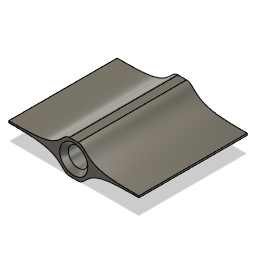
hose_to_balloon_symmetrical v2 (Autodesk Fusion 360 design; units mm, degrees)
Autodesk Fusion 360 part; units mm, degrees
sketch "Sketch1" plane through (0, 0, 0) normal (0, 0, 1) x (1, 0, 0)
  line L0 (15, -3.85) -> (-15, -3.85)
  line L1 (-15, -3.85) -> (-15, 3.85)
  line L2 (-15, 3.85) -> (15, 3.85)
  line L3 (15, 3.85) -> (15, -3.85)
  line L4 (15, -3.85) -> (-15, 3.85) construction
  line L5 (-15, -3.85) -> (15, 3.85) construction
  circle A0 centre (0, 0) radius 2.25
  line L6 (0, 2.25) -> (0, 3.85)
  dimension "d1" = 30
  dimension "d2" = 4.5
  dimension "d3" = 1.6
  constraint horizontal L0
  constraint perpendicular L0 L1
  constraint parallel L0 L2
  constraint parallel L1 L3
  constraint coincident L4 A0.centre
  constraint coincident L5 A0.centre
  constraint coincident A0.centre origin
  constraint coincident A0 L6.start
  constraint midpoint L2 L6.end
  constraint vertical L6
  measures "d1" distance of L0.start L0.end
  measures "d2" diameter of A0
  measures "d3" vertical distance of L6.start L6.end
extrude "Extrude1" add sketch "Sketch1" along normal blind 25
sketch "Sketch2" plane through (0, 0, 25) normal (0, 0, 1) x (1, 0, 0)
  circle A0 centre (0, 0) radius 2.25
  line L0 (15, 3.85) -> (-15, 3.85)
  line L1 (-15, 3.85) -> (-15, -3.85)
  line L2 (-15, -3.85) -> (15, -3.85)
  line L3 (15, -3.85) -> (15, 3.85)
  line L4 (-15, 0) -> (0, 0)
  line L5 (0, 0) -> (0, 3.85)
  line L6 (-15, 0.2) -> (-7, 0.2)
  line L7 (-7, 0.2) -> (-3.0262, 0.3362)
  line L8 (-3.0262, 0.3362) -> (-3, 3.85)
  line L9 (-3, 3.85) -> (-1, 3.85)
  spline S0 degree 4 poles (-15, 0.2) (-7, 0.2) (-3.0262, 0.3362) (-3, 3.85) (-1, 3.85) knots 0 0 0 0 0 1 1 1 1 1
  line L10 (-1, 3.85) -> (0, 3.85)
  dimension "d6" = 8
  dimension "d7" = 0.4
  dimension "d9" = 2
  dimension "d19" = 2
  constraint midpoint L1 L4.start
  constraint coincident A0.centre L4.end
  constraint midpoint L0 L5.end
  constraint coincident L1 L6.start
  constraint coincident L0 L8.end
  constraint horizontal L6
  constraint coincident L0 L9.end
  measures "d6" distance of L6.start L6.end
  measures "d9" distance of L8.end L9.end
extrude "Extrude2" cut sketch "Sketch2" against normal through all contours L0 L8 L9 S0 | L0 L1 L8 S0
mirror "Mirror1" about plane through (0, 0, 0) normal (0, 1, 0) of "Extrude2"
mirror "Mirror2" about plane through (0, 0, 0) normal (1, 0, 0) of "Extrude2", "Mirror1"
chamfer "Chamfer1" distance 1 angle 45 1 edges at (-2.0977, 0.8136, 25)
hole "Hole1" at (0, 0, 0) direction (0, 0, 1) diameter 5.8 depth 20 tip angle 118
equation "d4 = 25 mm"
equation "d16 = d4 - 5 mm"
named bodies: "hose_to_balloon"
